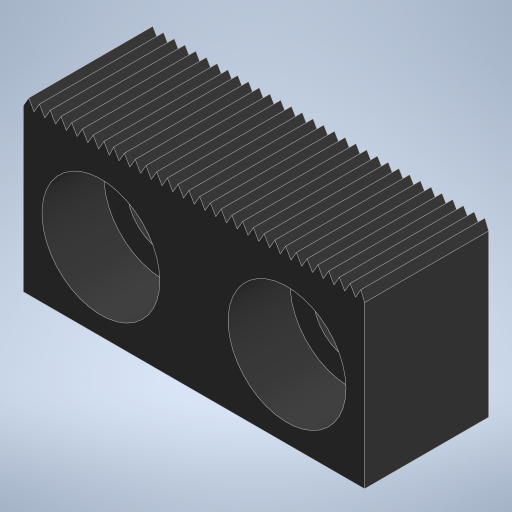
# Autodesk Inventor part: gripping_base
Saved by Autodesk Inventor 2024 (Build 280153000, 153)
## iProperties
Created: 2025-06-01
Part Number: gripping_base
Material: ゴム、黒
Document SubType Name: Modeling
Designer: 1412z
Density: 0.93 g/cm^3
Appearance: ゴム - 黒
Author: 1412z
Autodesk Inventor part; units mm, degrees
ref_plane "YZ Plane" through (0, 0, 0) normal (1, 0, 0) x (0, 1, 0)
ref_plane "XZ Plane" through (0, 0, 0) normal (0, 1, 0) x (-1, 0, 0)
ref_plane "XY Plane" through (0, 0, 0) normal (0, 0, 1) x (1, 0, 0)
sketch "スケッチ1" plane through (0, 0, 0) normal (0, 0, 1) x (1, 0, 0)
  line L0 (5, -2.5) -> (-5, -2.5)
  line L1 (-5, -2.5) -> (-5, 2.5)
  line L2 (-5, 2.5) -> (5, 2.5)
  line L3 (5, 2.5) -> (5, -2.5)
  line L4 (5, -2.5) -> (-5, 2.5) construction
  line L5 (-5, -2.5) -> (5, 2.5) construction
  circle A0 centre (-3, -0.5) radius 1.15
  circle A1 centre (3, -0.5) radius 1.15
  point P0 (0, 0)
  dimension "d0" = 10
  dimension "d1" = 5
  dimension "d2" = 2.3
  dimension "d3" = 2.3
  constraints: 12 end point, 2 centre point, 2 midpoint, 2 parallel, 1 horizontal, 1 perpendicular
  measures "d0" distance of L1.end L2.end
  measures "d1" distance of L0.end L1.end
  measures "d2" diameter of A0
  measures "d3" diameter of A1
extrude "押し出し1" add sketch "スケッチ1" along normal blind 4
sketch "スケッチ2" plane through (0, 0, 4) normal (0, 0, 1) x (1, 0, 0)
  circle A0 centre (-3, -0.5) radius 1.15 projected
  circle A1 centre (-3, -0.5) radius 1.9
  circle A2 centre (3, -0.5) radius 1.15 projected
  circle A3 centre (3, -0.5) radius 1.9
  point P0 (0, 0)
  dimension "d6" = 3.8
  dimension "d7" = 3.8
  constraints: 2 centre point, 2 coincident
  measures "d6" diameter of A1
  measures "d7" diameter of A3
extrude "押し出し2" cut sketch "スケッチ2" against normal blind 2
sketch "スケッチ3" plane through (-5, -2.5, 0) normal (0, -1, 0) x (1, 0, 0)
  line L0 (10, 0) -> (0, 0) projected
  line L1 (0, 0) -> (10, 0)
  line L2 (10, 0) -> (10, 4)
  line L3 (10, 4) -> (0, 4)
  line L4 (0, 4) -> (0, 0)
  point P0 (5, 0)
  constraints: 8 end point, 2 parallel, 1 horizontal, 1 perpendicular
extrude "押し出し3" add sketch "スケッチ3" along normal blind 0.5
sketch "スケッチ4" plane through (-5, 2.5, 0) normal (-1, 0, 0) x (0, 0, 1)
  line L0 (0, 0) -> (0, -5.5) projected
  line L1 (0, 0) -> (4, 0) projected
  line L2 (0, -5.5) -> (4, -5.5)
  line L3 (4, -5.5) -> (4, 0)
  line L4 (4, 0) -> (0, 0)
  line L5 (0, 0) -> (0, -5.5)
  point P0 (0, -2.5)
  constraints: 8 end point, 2 parallel, 1 horizontal, 1 perpendicular
extrude "押し出し4" add sketch "スケッチ4" along normal blind 0.5
sketch "スケッチ5" plane through (5, 2.5, 4) normal (1, 0, 0) x (0, 0, -1)
  line L0 (4, 0) -> (4, -5.5) projected
  line L1 (4, 0) -> (0, 0) projected
  line L2 (4, -5.5) -> (0, -5.5)
  line L3 (0, -5.5) -> (0, 0)
  line L4 (0, 0) -> (4, 0)
  line L5 (4, 0) -> (4, -5.5)
  point P0 (4, -2.5)
  constraints: 8 end point, 2 parallel, 1 horizontal, 1 perpendicular
extrude "押し出し5" add sketch "スケッチ5" along normal blind 0.5
sketch "スケッチ6" plane through (0, 0, 4) normal (0, 0, 1) x (1, 0, 0)
  line L0 (-5.5, 2.5) -> (5.5, 2.5) projected
  line L1 (-5.5, 2.5) -> (5.5, 2.5)
  line L2 (5.5, 2.5) -> (5.5, -3) projected
  line L3 (5.5, 2.5) -> (5.5, 2.2)
  line L4 (5.5, 2.2) -> (-5.5, 2.2)
  line L5 (-5.5, -3) -> (-5.5, 2.5) projected
  line L6 (-5.5, 2.2) -> (-5.5, 2.5)
  line L7 (-5.5, 2.2) -> (-5.3268, 2.5)
  line L8 (-5.5, 2.2) -> (-5.1536, 2.2) construction
  line L9 (-5.3268, 2.5) -> (-5.1536, 2.2)
  line L10 (-5.1536, 2.2) -> (-4.9804, 2.5)
  line L11 (-4.9804, 2.5) -> (-4.8072, 2.2)
  line L12 (-4.8072, 2.2) -> (-4.634, 2.5)
  line L13 (-4.634, 2.5) -> (-4.4608, 2.2)
  line L14 (-4.4608, 2.2) -> (-4.2876, 2.5)
  line L15 (-4.2876, 2.5) -> (-4.1144, 2.2)
  line L16 (-4.1144, 2.2) -> (-3.9412, 2.5)
  line L17 (-3.9412, 2.5) -> (-3.7679, 2.2)
  line L18 (-3.7679, 2.2) -> (-3.5947, 2.5)
  line L19 (-3.5947, 2.5) -> (-3.4215, 2.2)
  line L20 (-3.4215, 2.2) -> (-3.2483, 2.5)
  line L21 (-3.2483, 2.5) -> (-3.0751, 2.2)
  line L22 (-3.0751, 2.2) -> (-2.9019, 2.5)
  line L23 (-2.9019, 2.5) -> (-2.7287, 2.2)
  line L24 (-2.7287, 2.2) -> (-2.5869, 2.5)
  line L25 (-2.5869, 2.5) -> (-2.4137, 2.2)
  line L26 (-2.4137, 2.2) -> (-2.2405, 2.5)
  line L27 (-2.2405, 2.5) -> (-2.0673, 2.2)
  line L28 (-2.0673, 2.2) -> (-1.8941, 2.5)
  line L29 (-1.8941, 2.5) -> (-1.7209, 2.2)
  line L30 (-1.7209, 2.2) -> (-1.5477, 2.5)
  line L31 (-1.5477, 2.5) -> (-1.3745, 2.2)
  line L32 (-1.3745, 2.2) -> (-1.2012, 2.5)
  line L33 (-1.2012, 2.5) -> (-1.028, 2.2)
  line L34 (-1.028, 2.2) -> (-0.8548, 2.5)
  line L35 (-0.8548, 2.5) -> (-0.6816, 2.2)
  line L36 (-0.6816, 2.2) -> (-0.5084, 2.5)
  line L37 (-0.5084, 2.5) -> (-0.3352, 2.2)
  line L38 (-0.3352, 2.2) -> (-0.162, 2.5)
  line L39 (-0.162, 2.5) -> (0.0112, 2.2)
  line L40 (0.0112, 2.2) -> (0.1844, 2.5)
  line L41 (0.1844, 2.5) -> (0.3576, 2.2)
  line L42 (0.3576, 2.2) -> (0.5308, 2.5)
  line L43 (0.5308, 2.5) -> (0.704, 2.2)
  line L44 (0.704, 2.2) -> (0.8772, 2.5)
  line L45 (0.8772, 2.5) -> (1.0504, 2.2)
  line L46 (1.0504, 2.2) -> (1.2236, 2.5)
  line L47 (1.2236, 2.5) -> (1.3968, 2.2)
  line L48 (1.3968, 2.2) -> (1.57, 2.5)
  line L49 (1.57, 2.5) -> (1.7432, 2.2)
  line L50 (1.7432, 2.2) -> (1.9164, 2.5)
  line L51 (1.9164, 2.5) -> (2.0897, 2.2)
  line L52 (2.0897, 2.2) -> (2.2629, 2.5)
  line L53 (2.2629, 2.5) -> (2.4361, 2.2)
  line L54 (2.4361, 2.2) -> (2.6093, 2.5)
  line L55 (2.6093, 2.5) -> (2.7825, 2.2)
  line L56 (2.7825, 2.2) -> (2.9557, 2.5)
  line L57 (2.9557, 2.5) -> (3.1289, 2.2)
  line L58 (3.1289, 2.2) -> (3.3021, 2.5)
  line L59 (3.3021, 2.5) -> (3.4753, 2.2)
  line L60 (3.4753, 2.2) -> (3.6485, 2.5)
  line L61 (3.6485, 2.5) -> (3.8217, 2.2)
  line L62 (3.8217, 2.2) -> (3.9949, 2.5)
  line L63 (3.9949, 2.5) -> (4.1681, 2.2)
  line L64 (4.1681, 2.2) -> (4.3413, 2.5)
  line L65 (4.3413, 2.5) -> (4.5145, 2.2)
  line L66 (4.5145, 2.2) -> (4.6877, 2.5)
  line L67 (4.6877, 2.5) -> (4.8609, 2.2)
  line L68 (4.8609, 2.2) -> (5.0341, 2.5)
  line L69 (5.0341, 2.5) -> (5.2073, 2.2)
  line L70 (5.2073, 2.2) -> (5.3805, 2.5)
  line L71 (5.3805, 2.5) -> (5.5, 2.2)
  point P0 (0, 0)
  dimension "d16" = 0.3
  dimension "d17" = 60
  constraints: 134 end point, 54 parallel, 2 point on line, 1 collinear, 1 equal length, 1 horizontal, 70 other
  measures "d16" distance of L2.start L3.end
  measures "d17" angle of L8 L7
extrude "押し出し6" cut sketch "スケッチ6" against normal blind 10 contours L0 L7 L5 | L0 L10 L9 | L0 L12 L11 | L0 L14 L13 | L0 L16 L15 | L0 L18 L17 | L0 L20 L19 | L0 L22 L21 | L0 L24 L23 | L0 L26 L25 | L0 L28 L27 | L0 L30 L29 | L0 L32 L31 | L0 L34 L33 | L0 L36 L35 | L0 L38 L37 | L0 L40 L39 | L0 L42 L41 | L0 L44 L43 | L0 L46 L45 | L0 L48 L47 | L0 L50 L49 | L0 L52 L51 | L0 L54 L53 | L0 L56 L55 | L0 L58 L57 | L0 L60 L59 | L0 L62 L61 | L0 L64 L63 | L0 L66 L65 | L0 L68 L67 | L0 L70 L69 | L0 L2 L71
